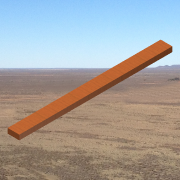
# Autodesk Inventor part: 2p2psh2
Saved by Autodesk Inventor 2014 SP1 (Build 180222100, 222)
## iProperties
Company: HERA Project
Created: 2013-09-03
Part Number: 2p2psh2
Material: Wood (Cherry)
Document SubType Name: Modeling
Designer: David DeBoer
Mass: 2056.37 g
Surface Area: 3183.04 cm^2
Volume: 4112.74 cm^3
Density: 0.5 g/cm^3
Description: pole stand support horizontal 2
Appearance: Cherry - Natural Low Gloss
Author: David DeBoer
Autodesk Inventor part; units mm, degrees
ref_plane "YZ Plane" through (0, 0, 0) normal (1, 0, 0) x (0, 1, 0)
ref_plane "XZ Plane" through (0, 0, 0) normal (0, 1, 0) x (-1, 0, 0)
ref_plane "XY Plane" through (0, 0, 0) normal (0, 0, 1) x (1, 0, 0)
sketch "Sketch1" plane through (0, 0, 0) normal (1, 0, 0) x (0, 1, 0)
  line L0 (0, 0) -> (38.1, 0)
  line L1 (38.1, 0) -> (38.1, -1168.4)
  line L2 (38.1, -1168.4) -> (0, -1168.4) construction
  line L3 (0, -1168.4) -> (0, 0)
  line L4 (0, -1168.4) -> (38.1, -1168.4)
  line L5 (0, -1168.4) -> (104.052, -1168.4) construction
  dimension "d0" = 38.1
  dimension "d1" = 1168.4
  dimension "d3" = 90
  constraints: 12 end point, 2 horizontal, 2 parallel, 1 perpendicular
  measures "d0" distance of L0.start L0.end
  measures "d1" distance of L2.end L0.start
  measures "d3" angle of L4 L3
extrude "Extrusion1" add sketch "Sketch1" along normal blind 88.9
body "Solid1"
